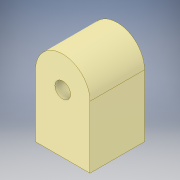
# Autodesk Inventor part: CLB_053_ScissorTopBarPlug
Saved by Autodesk Inventor 2018.3 (Build 223284000, 284)
## iProperties
Created: 2020-02-14
Part Number: CLB_053_ScissorTopBarPlug
Material: Nylon 6/6
Document SubType Name: Modeling
Designer: 22perngrac
Density: 1.13 g/cm^3
Appearance: Nylon 6
Author: 22perngrac
Autodesk Inventor part; units mm, degrees
ref_plane "YZ Plane" through (0, 0, 0) normal (1, 0, 0) x (0, 1, 0)
ref_plane "XZ Plane" through (0, 0, 0) normal (0, 1, 0) x (-1, 0, 0)
ref_plane "XY Plane" through (0, 0, 0) normal (0, 0, 1) x (1, 0, 0)
sketch "Sketch1" plane through (0, 0, 0) normal (0, 0, 1) x (1, 0, 0)
  line L0 (0, 0) -> (22.225, 0)
  line L1 (22.225, 0) -> (22.225, 25.4)
  line L2 (22.225, 25.4) -> (0, 25.4)
  line L3 (0, 25.4) -> (0, 0)
  arc A0 (22.225, 25.4) -> (0, 25.4) centre (11.1125, 25.4) ccw
  dimension "d0" = 25.4
  dimension "d1" = 22.225
  dimension "d4" = 11.1125
  constraints: 8 end point, 2 parallel, 2 point on circle, 2 tangent, 1 centre point, 1 horizontal, 1 perpendicular
  measures "d0" distance of L0.end L1.end
  measures "d1" distance of L1.end L2.end
  measures "d4" radius of A0
extrude "Extrusion2" add sketch "Sketch1" along normal blind 22.225
sketch "Sketch2" plane through (0, 0, 22.225) normal (0, 0, 1) x (1, 0, 0)
  line L0 (0, 0) -> (22.225, 0) projected
  line L1 (22.225, 0) -> (22.225, 25.4) projected
  point P0 (11.1125, 23.8252)
  dimension "d7" = 23.8252
  dimension "d8" = 11.1125
  measures "d7" distance from line of point (11.113, 23.825) L0
  measures "d8" distance from line of point (11.113, 23.825) L1
hole "Hole1" at (11.1125, 23.8252, 22.225) direction (0, 0, -1) diameter 6.35 end through all
body "Solid2"
